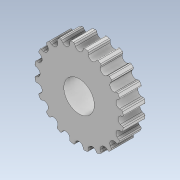
# Autodesk Inventor part: 2GT
Saved by Autodesk Inventor 2022 (Build 260153000, 153)
## iProperties
Created: 2023-05-02
Part Number: 2GT
Material: 一般
Document SubType Name: Modeling
Designer: JOU
Density: 1 g/cm^3
Appearance: 預設
Author: JOU
Autodesk Inventor part; units mm, degrees
ref_plane "YZ Plane" through (0, 0, 0) normal (1, 0, 0) x (0, 1, 0)
ref_plane "XZ Plane" through (0, 0, 0) normal (0, 1, 0) x (-1, 0, 0)
ref_plane "XY Plane" through (0, 0, 0) normal (0, 0, 1) x (1, 0, 0)
sketch "草圖1" plane through (0, 0, 0) normal (0, 0, 1) x (1, 0, 0)
  arc A0 (-0.7518, 6.0636) -> (-1.1588, 5.9991) centre (0, 0) ccw
  arc A1 (-1.1588, 5.9991) -> (-1.2788, 5.8304) centre (-1.1303, 5.8518) ccw
  arc A2 (-1.2782, 5.5484) -> (-1.2788, 5.8304) centre (-2.2685, 5.6874) ccw
  arc A3 (-2.2271, 5.24) -> (-1.2782, 5.5484) centre (-1.8278, 5.6255) ccw
  arc A4 (-2.3924, 5.4685) -> (-2.2271, 5.24) centre (-1.5077, 5.9346) ccw
  arc A5 (-2.3924, 5.4685) -> (-2.5887, 5.5345) centre (-2.5252, 5.3986) ccw
  arc A6 (-2.5887, 5.5345) -> (-2.9559, 5.3474) centre (0, 0) ccw
  arc A7 (-2.9559, 5.3474) -> (-3.0179, 5.1498) centre (-2.8833, 5.2161) ccw
  arc A8 (-2.9302, 4.8818) -> (-3.0179, 5.1498) centre (-3.915, 4.708) ccw
  arc A9 (-3.7374, 4.2953) -> (-2.9302, 4.8818) centre (-3.4767, 4.7853) ccw
  arc A10 (-3.9652, 4.4616) -> (-3.7374, 4.2953) centre (-3.2678, 5.1782) ccw
  arc A11 (-3.9652, 4.4616) -> (-4.1723, 4.4637) centre (-4.0698, 4.3541) ccw
  arc A12 (-4.1723, 4.4637) -> (-4.4637, 4.1723) centre (0, 0) ccw
  arc A13 (-4.4637, 4.1723) -> (-4.4616, 3.9652) centre (-4.3541, 4.0698) ccw
  arc A14 (-4.2953, 3.7374) -> (-4.4616, 3.9652) centre (-5.1782, 3.2678) ccw
  arc A15 (-4.8818, 2.9302) -> (-4.2953, 3.7374) centre (-4.7853, 3.4767) ccw
  arc A16 (-5.1498, 3.0179) -> (-4.8818, 2.9302) centre (-4.708, 3.915) ccw
  arc A17 (-5.1498, 3.0179) -> (-5.3474, 2.9559) centre (-5.2161, 2.8833) ccw
  arc A18 (-5.3474, 2.9559) -> (-5.5345, 2.5887) centre (0, 0) ccw
  arc A19 (-5.5345, 2.5887) -> (-5.4685, 2.3924) centre (-5.3986, 2.5252) ccw
  arc A20 (-5.24, 2.2271) -> (-5.4685, 2.3924) centre (-5.9346, 1.5077) ccw
  arc A21 (-5.5484, 1.2782) -> (-5.24, 2.2271) centre (-5.6255, 1.8278) ccw
  arc A22 (-5.8304, 1.2788) -> (-5.5484, 1.2782) centre (-5.6874, 2.2685) ccw
  arc A23 (-5.8304, 1.2788) -> (-5.9991, 1.1588) centre (-5.8518, 1.1303) ccw
  arc A24 (-5.9991, 1.1588) -> (-6.0636, 0.7518) centre (0, 0) ccw
  arc A25 (-6.0636, 0.7518) -> (-5.9402, 0.5855) centre (-5.9147, 0.7333) ccw
  arc A26 (-5.6718, 0.4989) -> (-5.9402, 0.5855) centre (-6.11, -0.4) ccw
  arc A27 (-5.6718, -0.4989) -> (-5.6718, 0.4989) centre (-5.915, 0) ccw
  arc A28 (-5.9402, -0.5855) -> (-5.6718, -0.4989) centre (-6.11, 0.4) ccw
  arc A29 (-5.9402, -0.5855) -> (-6.0636, -0.7518) centre (-5.9147, -0.7333) ccw
  arc A30 (-6.0636, -0.7518) -> (-5.9991, -1.1588) centre (0, 0) ccw
  arc A31 (-5.9991, -1.1588) -> (-5.8304, -1.2788) centre (-5.8518, -1.1303) ccw
  arc A32 (-5.5484, -1.2782) -> (-5.8304, -1.2788) centre (-5.6874, -2.2685) ccw
  arc A33 (-5.24, -2.2271) -> (-5.5484, -1.2782) centre (-5.6255, -1.8278) ccw
  arc A34 (-5.4685, -2.3924) -> (-5.24, -2.2271) centre (-5.9346, -1.5077) ccw
  arc A35 (-5.4685, -2.3924) -> (-5.5345, -2.5887) centre (-5.3986, -2.5252) ccw
  arc A36 (-5.5345, -2.5887) -> (-5.3474, -2.9559) centre (0, 0) ccw
  arc A37 (-5.3474, -2.9559) -> (-5.1498, -3.0179) centre (-5.2161, -2.8833) ccw
  arc A38 (-4.8818, -2.9302) -> (-5.1498, -3.0179) centre (-4.708, -3.915) ccw
  arc A39 (-4.2953, -3.7374) -> (-4.8818, -2.9302) centre (-4.7853, -3.4767) ccw
  arc A40 (-4.4616, -3.9652) -> (-4.2953, -3.7374) centre (-5.1782, -3.2678) ccw
  arc A41 (-4.4616, -3.9652) -> (-4.4637, -4.1723) centre (-4.3541, -4.0698) ccw
  arc A42 (-4.4637, -4.1723) -> (-4.1723, -4.4637) centre (0, 0) ccw
  arc A43 (-4.1723, -4.4637) -> (-3.9652, -4.4616) centre (-4.0698, -4.3541) ccw
  arc A44 (-3.7374, -4.2953) -> (-3.9652, -4.4616) centre (-3.2678, -5.1782) ccw
  arc A45 (-2.9302, -4.8818) -> (-3.7374, -4.2953) centre (-3.4767, -4.7853) ccw
  arc A46 (-3.0179, -5.1498) -> (-2.9302, -4.8818) centre (-3.915, -4.708) ccw
  arc A47 (-3.0179, -5.1498) -> (-2.9559, -5.3474) centre (-2.8833, -5.2161) ccw
  arc A48 (-2.9559, -5.3474) -> (-2.5887, -5.5345) centre (0, 0) ccw
  arc A49 (-2.5887, -5.5345) -> (-2.3924, -5.4685) centre (-2.5252, -5.3986) ccw
  arc A50 (-2.2271, -5.24) -> (-2.3924, -5.4685) centre (-1.5077, -5.9346) ccw
  arc A51 (-1.2782, -5.5484) -> (-2.2271, -5.24) centre (-1.8278, -5.6255) ccw
  arc A52 (-1.2788, -5.8304) -> (-1.2782, -5.5484) centre (-2.2685, -5.6874) ccw
  arc A53 (-1.2788, -5.8304) -> (-1.1588, -5.9991) centre (-1.1303, -5.8518) ccw
  arc A54 (-1.1588, -5.9991) -> (-0.7518, -6.0636) centre (0, 0) ccw
  arc A55 (-0.7518, -6.0636) -> (-0.5855, -5.9402) centre (-0.7333, -5.9147) ccw
  arc A56 (-0.4989, -5.6718) -> (-0.5855, -5.9402) centre (0.4, -6.11) ccw
  arc A57 (0.4989, -5.6718) -> (-0.4989, -5.6718) centre (0, -5.915) ccw
  arc A58 (0.5855, -5.9402) -> (0.4989, -5.6718) centre (-0.4, -6.11) ccw
  arc A59 (0.5855, -5.9402) -> (0.7518, -6.0636) centre (0.7333, -5.9147) ccw
  arc A60 (0.7518, -6.0636) -> (1.1588, -5.9991) centre (0, 0) ccw
  arc A61 (1.1588, -5.9991) -> (1.2788, -5.8304) centre (1.1303, -5.8518) ccw
  arc A62 (1.2782, -5.5484) -> (1.2788, -5.8304) centre (2.2685, -5.6874) ccw
  arc A63 (2.2271, -5.24) -> (1.2782, -5.5484) centre (1.8278, -5.6255) ccw
  arc A64 (2.3924, -5.4685) -> (2.2271, -5.24) centre (1.5077, -5.9346) ccw
  arc A65 (2.3924, -5.4685) -> (2.5887, -5.5345) centre (2.5252, -5.3986) ccw
  arc A66 (2.5887, -5.5345) -> (2.9559, -5.3474) centre (0, 0) ccw
  arc A67 (2.9559, -5.3474) -> (3.0179, -5.1498) centre (2.8833, -5.2161) ccw
  arc A68 (2.9302, -4.8818) -> (3.0179, -5.1498) centre (3.915, -4.708) ccw
  arc A69 (3.7374, -4.2953) -> (2.9302, -4.8818) centre (3.4767, -4.7853) ccw
  arc A70 (3.9652, -4.4616) -> (3.7374, -4.2953) centre (3.2678, -5.1782) ccw
  arc A71 (3.9652, -4.4616) -> (4.1723, -4.4637) centre (4.0698, -4.3541) ccw
  arc A72 (4.1723, -4.4637) -> (4.4637, -4.1723) centre (0, 0) ccw
  arc A73 (4.4637, -4.1723) -> (4.4616, -3.9652) centre (4.3541, -4.0698) ccw
  arc A74 (4.2953, -3.7374) -> (4.4616, -3.9652) centre (5.1782, -3.2678) ccw
  arc A75 (4.8818, -2.9302) -> (4.2953, -3.7374) centre (4.7853, -3.4767) ccw
  arc A76 (5.1498, -3.0179) -> (4.8818, -2.9302) centre (4.708, -3.915) ccw
  arc A77 (5.1498, -3.0179) -> (5.3474, -2.9559) centre (5.2161, -2.8833) ccw
  arc A78 (5.3474, -2.9559) -> (5.5345, -2.5887) centre (0, 0) ccw
  arc A79 (5.5345, -2.5887) -> (5.4685, -2.3924) centre (5.3986, -2.5252) ccw
  arc A80 (5.24, -2.2271) -> (5.4685, -2.3924) centre (5.9346, -1.5077) ccw
  arc A81 (5.5484, -1.2782) -> (5.24, -2.2271) centre (5.6255, -1.8278) ccw
  arc A82 (5.8304, -1.2788) -> (5.5484, -1.2782) centre (5.6874, -2.2685) ccw
  arc A83 (5.8304, -1.2788) -> (5.9991, -1.1588) centre (5.8518, -1.1303) ccw
  arc A84 (5.9991, -1.1588) -> (6.0636, -0.7518) centre (0, 0) ccw
  arc A85 (6.0636, -0.7518) -> (5.9402, -0.5855) centre (5.9147, -0.7333) ccw
  arc A86 (5.6718, -0.4989) -> (5.9402, -0.5855) centre (6.11, 0.4) ccw
  arc A87 (5.6718, 0.4989) -> (5.6718, -0.4989) centre (5.915, 0) ccw
  arc A88 (5.9402, 0.5855) -> (5.6718, 0.4989) centre (6.11, -0.4) ccw
  arc A89 (5.9402, 0.5855) -> (6.0636, 0.7518) centre (5.9147, 0.7333) ccw
  arc A90 (6.0636, 0.7518) -> (5.9991, 1.1588) centre (0, 0) ccw
  arc A91 (5.9991, 1.1588) -> (5.8304, 1.2788) centre (5.8518, 1.1303) ccw
  arc A92 (5.5484, 1.2782) -> (5.8304, 1.2788) centre (5.6874, 2.2685) ccw
  arc A93 (5.24, 2.2271) -> (5.5484, 1.2782) centre (5.6255, 1.8278) ccw
  arc A94 (5.4685, 2.3924) -> (5.24, 2.2271) centre (5.9346, 1.5077) ccw
  arc A95 (5.4685, 2.3924) -> (5.5345, 2.5887) centre (5.3986, 2.5252) ccw
  arc A96 (5.5345, 2.5887) -> (5.3474, 2.9559) centre (0, 0) ccw
  arc A97 (5.3474, 2.9559) -> (5.1498, 3.0179) centre (5.2161, 2.8833) ccw
  arc A98 (4.8818, 2.9302) -> (5.1498, 3.0179) centre (4.708, 3.915) ccw
  arc A99 (4.2953, 3.7374) -> (4.8818, 2.9302) centre (4.7853, 3.4767) ccw
  arc A100 (4.4616, 3.9652) -> (4.2953, 3.7374) centre (5.1782, 3.2678) ccw
  arc A101 (4.4616, 3.9652) -> (4.4637, 4.1723) centre (4.3541, 4.0698) ccw
  arc A102 (4.4637, 4.1723) -> (4.1723, 4.4637) centre (0, 0) ccw
  arc A103 (4.1723, 4.4637) -> (3.9652, 4.4616) centre (4.0698, 4.3541) ccw
  arc A104 (3.7374, 4.2953) -> (3.9652, 4.4616) centre (3.2678, 5.1782) ccw
  arc A105 (2.9302, 4.8818) -> (3.7374, 4.2953) centre (3.4767, 4.7853) ccw
  arc A106 (3.0179, 5.1498) -> (2.9302, 4.8818) centre (3.915, 4.708) ccw
  arc A107 (3.0179, 5.1498) -> (2.9559, 5.3474) centre (2.8833, 5.2161) ccw
  arc A108 (2.9559, 5.3474) -> (2.5887, 5.5345) centre (0, 0) ccw
  arc A109 (2.5887, 5.5345) -> (2.3924, 5.4685) centre (2.5252, 5.3986) ccw
  arc A110 (2.2271, 5.24) -> (2.3924, 5.4685) centre (1.5077, 5.9346) ccw
  arc A111 (1.2782, 5.5484) -> (2.2271, 5.24) centre (1.8278, 5.6255) ccw
  arc A112 (1.2788, 5.8304) -> (1.2782, 5.5484) centre (2.2685, 5.6874) ccw
  arc A113 (1.2788, 5.8304) -> (1.1588, 5.9991) centre (1.1303, 5.8518) ccw
  arc A114 (1.1588, 5.9991) -> (0.7518, 6.0636) centre (0, 0) ccw
  arc A115 (0.7518, 6.0636) -> (0.5855, 5.9402) centre (0.7333, 5.9147) ccw
  arc A116 (0.4989, 5.6718) -> (0.5855, 5.9402) centre (-0.4, 6.11) ccw
  arc A117 (-0.4989, 5.6718) -> (0.4989, 5.6718) centre (0, 5.915) ccw
  arc A118 (-0.5855, 5.9402) -> (-0.4989, 5.6718) centre (0.4, 6.11) ccw
  arc A119 (-0.5855, 5.9402) -> (-0.7518, 6.0636) centre (-0.7333, 5.9147) ccw
  circle A120 centre (0, 0) radius 2.1
  dimension "d0" = 4.2
  constraints: 240 point on circle, 121 centre point, 1 coincident, 362 other
  measures "d0" diameter of A120
extrude "擠出1" add sketch "草圖1" along normal blind 3
sketch "草圖2" plane through (0, 0, 0) normal (0, 0, -1) x (-1, 0, 0)
  point P0 (0, 0)
